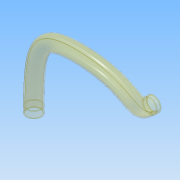
# Autodesk Inventor part: Top_Front Pipe 4
Saved by Autodesk Inventor 2018.1 (Build 221171000, 171)
## iProperties
Created: 2019-03-21
Part Number: Top_Front Pipe 4
Material: PMMA Plastic
Document SubType Name: Modeling
Designer: James
Density: 1.188 g/cm^3
Appearance: Clear - Yellow
Author: James
Autodesk Inventor part; units mm, degrees
ref_plane "YZ Plane" through (0, 0, 0) normal (1, 0, 0) x (0, 1, 0)
ref_plane "XZ Plane" through (0, 0, 0) normal (0, 1, 0) x (-1, 0, 0)
ref_plane "XY Plane" through (0, 0, 0) normal (0, 0, 1) x (1, 0, 0)
sketch "Sketch1" plane through (0, 0, 0) normal (0, 1, 0) x (-1, 0, 0)
  circle A0 centre (0, 0) radius 23
  circle A1 centre (0, 0) radius 20
  dimension "d0" = 3
  dimension "d1" = 40
  constraints: 2 centre point, 2 coincident
  measures "d0" radial gap between concentric circles of A0 A1
  measures "d1" diameter of A1
extrude "Extrusion1" add sketch "Sketch1" along normal blind 12
sketch "Sketch2" plane through (0, 0, 0) normal (0, 0, 1) x (1, 0, 0)
  line L0 (23, 12) -> (-23, 12) projected
  point P0 (0, 0)
  point P1 (0, 5)
  point P2 (0, 12)
  dimension "d4" = 7
  constraints: 1 midpoint, 1 vertical alignment
  measures "d4" distance from line of L0 point (0, 5)
hole "Hole1" at (0, 5, 0) direction (0, 0, -1) diameter 4.5 end through all
sketch "Sketch3" plane through (0, 0, 0) normal (0, -1, 0) x (1, 0, 0)
  circle A0 centre (0, 0) radius 20 projected
  circle A1 centre (0, 0) radius 23 projected
sketch3d "3D Sketch1"
  spline S0 degree 4 poles (0, 0, 0) (0, -44.5, 0) (0, -44.5, 90) (-272.5, -44.5, 90) (-272.5, -85.5, 90) (-272.5, -85.5, -92) knots 1 1 1 1 1 2 3 3 3 3 3
  dimension "d21" = 44.5
  dimension "d22" = 90
  dimension "d23" = 272.5
  dimension "d24" = 41
  dimension "d25" = 182
sweep "Sweep1" add profiles "Sketch3" path "3D Sketch1"
sketch "Sketch4" plane through (-272.5, -85.5, -92) normal (0, 0, -1) x (-1, 0, 0)
  spline S0 degree 6 poles (11.1809, -16.5828) (-16.3721, -35.1603) (-43.2999, -3.7576) (-30.7375, 45.588) (19.7184, 38.7322) (38.7339, 1.9947) (11.1809, -16.5828) knots 0 0 0 0 0 0 0 1 1 1 1 1 1 1 weights 1.669078 1.03673 1.038347 0.853534 1.038347 1.03673 1.669078 projected
  circle A0 centre (0, 0) radius 23 projected
  point P0 (-272.5, 85.5)
  point P1 (13.147, -18.8721)
  constraints: 2 other
extrude "Extrusion2" add sketch "Sketch4" along normal blind 20 contours S0 picked at (4.4973, -21.3909)
body "Solid1"
